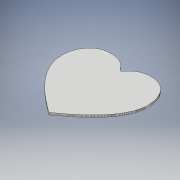
# Autodesk Inventor part: pcb
Saved by Autodesk Inventor 2018 (Build 220112000, 112)
## iProperties
Created: 2020-01-18
Part Number: pcb
Material: Generic
Document SubType Name: Modeling
Designer: Lorenzo Spadaro
Density: 1 g/cm^3
Appearance: Default
Author: Lorenzo Spadaro
Autodesk Inventor part; units mm, degrees
ref_plane "YZ Plane" through (0, 0, 0) normal (1, 0, 0) x (0, 1, 0)
ref_plane "XZ Plane" through (0, 0, 0) normal (0, 1, 0) x (-1, 0, 0)
ref_plane "XY Plane" through (0, 0, 0) normal (0, 0, 1) x (1, 0, 0)
sketch "Sketch1" plane through (0, 0, 0) normal (0, 0, 1) x (1, 0, 0)
  line L0 (-17.245, 29.3528) -> (-16.8785, 29.3804)
  line L1 (-16.8785, 29.3804) -> (-14.6595, 29.4537)
  line L2 (-14.6595, 29.4537) -> (-13.1751, 29.3976)
  line L3 (-13.1751, 29.3976) -> (-12.0678, 29.2897)
  line L4 (-12.0678, 29.2897) -> (-10.9712, 29.1184)
  line L5 (-10.9712, 29.1184) -> (-10.2487, 28.9658)
  line L6 (-10.2487, 28.9658) -> (-9.5347, 28.7803)
  line L7 (-9.5347, 28.7803) -> (-8.8307, 28.56)
  line L8 (-8.8307, 28.56) -> (-8.1383, 28.3029)
  line L9 (-8.1383, 28.3029) -> (-7.459, 28.0073)
  line L10 (-7.459, 28.0073) -> (-6.7943, 27.6713)
  line L11 (-6.7943, 27.6713) -> (-6.5134, 27.52)
  line L12 (-6.5134, 27.52) -> (-5.6972, 27.03)
  line L13 (-5.6972, 27.03) -> (-4.6649, 26.2999)
  line L14 (-4.6649, 26.2999) -> (-3.4534, 25.2847)
  line L15 (-3.4534, 25.2847) -> (0.0159, 21.5885)
  line L16 (0.0159, 21.5885) -> (3.8507, 25.6083)
  line L17 (3.8507, 25.6083) -> (5.228, 26.6918)
  line L18 (5.228, 26.6918) -> (6.211, 27.3322)
  line L19 (6.211, 27.3322) -> (6.5543, 27.5333)
  line L20 (6.5543, 27.5333) -> (6.9023, 27.7227)
  line L21 (6.9023, 27.7227) -> (7.2549, 27.9007)
  line L22 (7.2549, 27.9007) -> (7.6118, 28.0676)
  line L23 (7.6118, 28.0676) -> (7.9727, 28.2236)
  line L24 (7.9727, 28.2236) -> (8.7059, 28.504)
  line L25 (8.7059, 28.504) -> (9.4527, 28.7439)
  line L26 (9.4527, 28.7439) -> (10.2112, 28.9453)
  line L27 (10.2112, 28.9453) -> (10.9798, 29.1102)
  line L28 (10.9798, 29.1102) -> (11.7563, 29.2404)
  line L29 (11.7563, 29.2404) -> (12.539, 29.3382)
  line L30 (12.539, 29.3382) -> (13.7207, 29.4281)
  line L31 (13.7207, 29.4281) -> (15.3008, 29.4526)
  line L32 (15.3008, 29.4526) -> (17.2627, 29.3524)
  line L33 (17.2627, 29.3524) -> (17.6451, 29.3169)
  line L34 (17.6451, 29.3169) -> (18.0256, 29.2698)
  line L35 (18.0256, 29.2698) -> (18.4039, 29.2117)
  line L36 (18.4039, 29.2117) -> (19.1535, 29.0627)
  line L37 (19.1535, 29.0627) -> (19.8923, 28.8712)
  line L38 (19.8923, 28.8712) -> (20.6192, 28.6391)
  line L39 (20.6192, 28.6391) -> (21.3326, 28.3678)
  line L40 (21.3326, 28.3678) -> (22.0311, 28.0591)
  line L41 (22.0311, 28.0591) -> (22.7133, 27.7144)
  line L42 (22.7133, 27.7144) -> (23.3776, 27.3355)
  line L43 (23.3776, 27.3355) -> (24.0229, 26.9239)
  line L44 (24.0229, 26.9239) -> (24.6476, 26.4813)
  line L45 (24.6476, 26.4813) -> (25.2503, 26.0093)
  line L46 (25.2503, 26.0093) -> (25.8295, 25.5093)
  line L47 (25.8295, 25.5093) -> (26.384, 24.9833)
  line L48 (26.384, 24.9833) -> (26.9121, 24.4326)
  line L49 (26.9121, 24.4326) -> (27.2277, 24.0852)
  line L50 (27.2277, 24.0852) -> (27.5326, 23.7298)
  line L51 (27.5326, 23.7298) -> (27.8268, 23.3666)
  line L52 (27.8268, 23.3666) -> (28.1103, 22.996)
  line L53 (28.1103, 22.996) -> (28.3833, 22.6181)
  line L54 (28.3833, 22.6181) -> (28.646, 22.2334)
  line L55 (28.646, 22.2334) -> (28.8982, 21.842)
  line L56 (28.8982, 21.842) -> (29.1402, 21.4444)
  line L57 (29.1402, 21.4444) -> (29.3721, 21.0406)
  line L58 (29.3721, 21.0406) -> (29.5938, 20.6312)
  line L59 (29.5938, 20.6312) -> (29.8055, 20.2163)
  line L60 (29.8055, 20.2163) -> (30.1993, 19.3715)
  line L61 (30.1993, 19.3715) -> (30.5539, 18.5084)
  line L62 (30.5539, 18.5084) -> (30.8702, 17.6295)
  line L63 (30.8702, 17.6295) -> (31.1488, 16.7371)
  line L64 (31.1488, 16.7371) -> (31.3903, 15.8335)
  line L65 (31.3903, 15.8335) -> (31.5955, 14.921)
  line L66 (31.5955, 14.921) -> (31.765, 14.0021)
  line L67 (31.765, 14.0021) -> (31.8995, 13.079)
  line L68 (31.8995, 13.079) -> (31.9996, 12.1541)
  line L69 (31.9996, 12.1541) -> (31.9996, 8.1022)
  line L70 (31.9996, 8.1022) -> (31.9394, 7.5177)
  line L71 (31.9394, 7.5177) -> (31.865, 6.9326)
  line L72 (31.865, 6.9326) -> (31.777, 6.3504)
  line L73 (31.777, 6.3504) -> (31.6758, 5.7711)
  line L74 (31.6758, 5.7711) -> (31.5617, 5.1948)
  line L75 (31.5617, 5.1948) -> (31.435, 4.6216)
  line L76 (31.435, 4.6216) -> (31.296, 4.0515)
  line L77 (31.296, 4.0515) -> (31.1451, 3.4847)
  line L78 (31.1451, 3.4847) -> (30.9824, 2.9211)
  line L79 (30.9824, 2.9211) -> (30.8085, 2.3608)
  line L80 (30.8085, 2.3608) -> (30.6235, 1.8039)
  line L81 (30.6235, 1.8039) -> (30.2216, 0.7006)
  line L82 (30.2216, 0.7006) -> (29.7794, -0.3882)
  line L83 (29.7794, -0.3882) -> (29.2993, -1.462)
  line L84 (29.2993, -1.462) -> (28.7838, -2.5204)
  line L85 (28.7838, -2.5204) -> (28.2354, -3.5627)
  line L86 (28.2354, -3.5627) -> (27.6567, -4.5884)
  line L87 (27.6567, -4.5884) -> (26.7372, -6.0947)
  line L88 (26.7372, -6.0947) -> (25.7634, -7.5606)
  line L89 (25.7634, -7.5606) -> (25.2678, -8.2596)
  line L90 (25.2678, -8.2596) -> (24.7624, -8.9506)
  line L91 (24.7624, -8.9506) -> (24.2476, -9.6339)
  line L92 (24.2476, -9.6339) -> (23.7235, -10.3096)
  line L93 (23.7235, -10.3096) -> (23.1905, -10.9779)
  line L94 (23.1905, -10.9779) -> (22.099, -12.2928)
  line L95 (22.099, -12.2928) -> (20.9751, -13.5799)
  line L96 (20.9751, -13.5799) -> (19.8211, -14.8405)
  line L97 (19.8211, -14.8405) -> (18.6393, -16.0758)
  line L98 (18.6393, -16.0758) -> (17.4319, -17.2871)
  line L99 (17.4319, -17.2871) -> (15.5777, -19.0618)
  line L100 (15.5777, -19.0618) -> (13.6785, -20.7898)
  line L101 (13.6785, -20.7898) -> (10.4337, -23.5772)
  line L102 (10.4337, -23.5772) -> (8.4513, -25.2013)
  line L103 (8.4513, -25.2013) -> (0.0167, -31.499)
  line L104 (0.0167, -31.499) -> (-4.465, -28.2383)
  line L105 (-4.465, -28.2383) -> (-7.1134, -26.2189)
  line L106 (-7.1134, -26.2189) -> (-8.8556, -24.8418)
  line L107 (-8.8556, -24.8418) -> (-10.5755, -23.4377)
  line L108 (-10.5755, -23.4377) -> (-12.27, -22.0042)
  line L109 (-12.27, -22.0042) -> (-13.936, -20.5394)
  line L110 (-13.936, -20.5394) -> (-14.7574, -19.7945)
  line L111 (-14.7574, -19.7945) -> (-15.5704, -19.0409)
  line L112 (-15.5704, -19.0409) -> (-16.3748, -18.2784)
  line L113 (-16.3748, -18.2784) -> (-17.1701, -17.5067)
  line L114 (-17.1701, -17.5067) -> (-17.956, -16.7255)
  line L115 (-17.956, -16.7255) -> (-18.7321, -15.9345)
  line L116 (-18.7321, -15.9345) -> (-19.4979, -15.1335)
  line L117 (-19.4979, -15.1335) -> (-20.2531, -14.3223)
  line L118 (-20.2531, -14.3223) -> (-20.9973, -13.5005)
  line L119 (-20.9973, -13.5005) -> (-21.7301, -12.6678)
  line L120 (-21.7301, -12.6678) -> (-22.4512, -11.8241)
  line L121 (-22.4512, -11.8241) -> (-23.1601, -10.969)
  line L122 (-23.1601, -10.969) -> (-23.8564, -10.1022)
  line L123 (-23.8564, -10.1022) -> (-24.7026, -8.9915)
  line L124 (-24.7026, -8.9915) -> (-25.5224, -7.8556)
  line L125 (-25.5224, -7.8556) -> (-26.3122, -6.6953)
  line L126 (-26.3122, -6.6953) -> (-27.068, -5.5112)
  line L127 (-27.068, -5.5112) -> (-27.4321, -4.9103)
  line L128 (-27.4321, -4.9103) -> (-27.7862, -4.3037)
  line L129 (-27.7862, -4.3037) -> (-28.13, -3.6914)
  line L130 (-28.13, -3.6914) -> (-28.4628, -3.0735)
  line L131 (-28.4628, -3.0735) -> (-28.7844, -2.4501)
  line L132 (-28.7844, -2.4501) -> (-29.0942, -1.8212)
  line L133 (-29.0942, -1.8212) -> (-29.3916, -1.1869)
  line L134 (-29.3916, -1.1869) -> (-29.6764, -0.5473)
  line L135 (-29.6764, -0.5473) -> (-29.9478, 0.0975)
  line L136 (-29.9478, 0.0975) -> (-30.2056, 0.7476)
  line L137 (-30.2056, 0.7476) -> (-30.4492, 1.4027)
  line L138 (-30.4492, 1.4027) -> (-30.6781, 2.0629)
  line L139 (-30.6781, 2.0629) -> (-30.8919, 2.728)
  line L140 (-30.8919, 2.728) -> (-31.0901, 3.398)
  line L141 (-31.0901, 3.398) -> (-31.2721, 4.0728)
  line L142 (-31.2721, 4.0728) -> (-31.4376, 4.7523)
  line L143 (-31.4376, 4.7523) -> (-31.5861, 5.4366)
  line L144 (-31.5861, 5.4366) -> (-31.7171, 6.1254)
  line L145 (-31.7171, 6.1254) -> (-31.83, 6.8188)
  line L146 (-31.83, 6.8188) -> (-31.9245, 7.5166)
  line L147 (-31.9245, 7.5166) -> (-32, 8.2188)
  line L148 (-32, 8.2188) -> (-32, 11.9121)
  line L149 (-32, 11.9121) -> (-31.867, 13.1401)
  line L150 (-31.867, 13.1401) -> (-31.6762, 14.3631)
  line L151 (-31.6762, 14.3631) -> (-31.4255, 15.576)
  line L152 (-31.4255, 15.576) -> (-31.1126, 16.7738)
  line L153 (-31.1126, 16.7738) -> (-30.7354, 17.9518)
  line L154 (-30.7354, 17.9518) -> (-30.4471, 18.7236)
  line L155 (-30.4471, 18.7236) -> (-30.1287, 19.4829)
  line L156 (-30.1287, 19.4829) -> (-29.7794, 20.2281)
  line L157 (-29.7794, 20.2281) -> (-29.3986, 20.958)
  line L158 (-29.3986, 20.958) -> (-28.9857, 21.6709)
  line L159 (-28.9857, 21.6709) -> (-28.54, 22.3654)
  line L160 (-28.54, 22.3654) -> (-28.0609, 23.0401)
  line L161 (-28.0609, 23.0401) -> (-27.7919, 23.3924)
  line L162 (-27.7919, 23.3924) -> (-27.5134, 23.738)
  line L163 (-27.5134, 23.738) -> (-27.2255, 24.0766)
  line L164 (-27.2255, 24.0766) -> (-26.9284, 24.4079)
  line L165 (-26.9284, 24.4079) -> (-26.6224, 24.7316)
  line L166 (-26.6224, 24.7316) -> (-26.3078, 25.0474)
  line L167 (-26.3078, 25.0474) -> (-25.9848, 25.3548)
  line L168 (-25.9848, 25.3548) -> (-25.6537, 25.6537)
  line L169 (-25.6537, 25.6537) -> (-25.3146, 25.9436)
  line L170 (-25.3146, 25.9436) -> (-24.9678, 26.2242)
  line L171 (-24.9678, 26.2242) -> (-24.6136, 26.4952)
  line L172 (-24.6136, 26.4952) -> (-24.2523, 26.7562)
  line L173 (-24.2523, 26.7562) -> (-23.8839, 27.007)
  line L174 (-23.8839, 27.007) -> (-23.5089, 27.2472)
  line L175 (-23.5089, 27.2472) -> (-23.1275, 27.4764)
  line L176 (-23.1275, 27.4764) -> (-22.7397, 27.6944)
  line L177 (-22.7397, 27.6944) -> (-22.346, 27.9008)
  line L178 (-22.346, 27.9008) -> (-21.9466, 28.0952)
  line L179 (-21.9466, 28.0952) -> (-21.5418, 28.2774)
  line L180 (-21.5418, 28.2774) -> (-21.1317, 28.4471)
  line L181 (-21.1317, 28.4471) -> (-20.7166, 28.6038)
  line L182 (-20.7166, 28.6038) -> (-20.2967, 28.7472)
  line L183 (-20.2967, 28.7472) -> (-19.8724, 28.8771)
  line L184 (-19.8724, 28.8771) -> (-19.4437, 28.9931)
  line L185 (-19.4437, 28.9931) -> (-19.011, 29.0949)
  line L186 (-19.011, 29.0949) -> (-18.5745, 29.182)
  line L187 (-18.5745, 29.182) -> (-18.1346, 29.2543)
  line L188 (-18.1346, 29.2543) -> (-17.6913, 29.3114)
  line L189 (-17.6913, 29.3114) -> (-17.245, 29.3528)
  point P0 (0, 0)
  constraints: 380 end point, 3 perpendicular, 1 parallel
extrude "Extrusion1" add sketch "Sketch1" along normal blind 1.6
body "Solid1"
